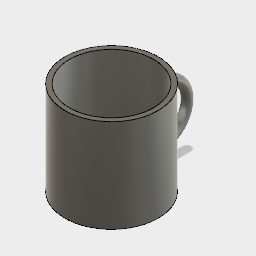
茶杯 (Autodesk Fusion 360 design; units mm, degrees)
Autodesk Fusion 360 part; units mm, degrees
cylinder "圆柱体基本要素1" add diameter 20 height 20 placed x (1, 0, 0) y (0, 0, -1) z (0, 1, 0) at (0, 0, 0) makes body 1
form "造型1" [no effect]
cylinder "圆柱体基本要素2" add diameter 18 height 20 placed x (1, 0, 0) y (0, 0, -1) z (0, 1, 0) at (0, 0, 40) separate body makes body 2
torus "圆环体基本要素1" add centre line diameter 12 section diameter 2 placed x (1, 0, 0) y (0, 0, -1) z (0, 1, 0) at (0, 0, -60) separate body makes body 3
move_body "MoveFace1" bodies 3 to x (0, -1, 0) y (1, 0, 0) z (0, 0, 1) at (0.1266, 9.2888, 49.9503) on bodies 3
combine "合并1" operation add target body 1 tool bodies 3
move_body "对齐1" bodies 2 to x (1, 0, 0) y (0, 1, 0) z (0, 0, 1) at (0, 0, 0)
move_body "对齐2" bodies 1 to x (1, 0, 0) y (0, 1, 0) z (0, 0, 1) at (0, 0, 40)
move_face "偏移面1" offset -2 1 faces at (1.5, 0, 37.9071) on bodies 2
combine "合并2" operation cut target body 1 tool bodies 2
